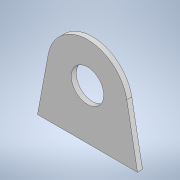
# Autodesk Inventor part: 76. Стопор штуцера
Saved by Autodesk Inventor 2021 (Build 250183000, 183)
## iProperties
Created: 2021-03-15
Part Number: 76. Стопор штуцера
Material: Типовые
Document SubType Name: Modeling
Designer: Данил
Density: 1 g/cm^3
Appearance: По умолчанию
Author: Данил
Autodesk Inventor part; units mm, degrees
ref_plane "YZ Plane" through (0, 0, 0) normal (1, 0, 0) x (0, 1, 0)
ref_plane "XZ Plane" through (0, 0, 0) normal (0, 1, 0) x (-1, 0, 0)
ref_plane "XY Plane" through (0, 0, 0) normal (0, 0, 1) x (1, 0, 0)
sketch "Эскиз1" plane through (0, 0, 0) normal (0, 0, 1) x (1, 0, 0)
  line L0 (0, 9) -> (0, -9) construction
  line L1 (0, -9) -> (10, -9)
  arc A0 (0, -2.25) -> (0, 4.25) centre (0, 1) ccw
  arc A1 (7.8648, 2.4648) -> (0, 9) centre (0, 1) ccw
  line L2 (7.8648, 2.4648) -> (10, -9)
  line L3 (0, 9) -> (0, 4.25)
  line L4 (0, -2.25) -> (0, -9)
  point P0 (0, 0)
  point P1 (0, 0)
  dimension "d0" = 18
  dimension "d1" = 10
  dimension "d2" = 3.25
  dimension "d3" = 10
  constraints: 10 end point, 4 point on circle, 3 point on line, 2 centre point, 2 coincident, 2 collinear, 1 horizontal, 1 midpoint, 1 tangent, 1 vertical
  measures "d0" distance of L0.start L0.end
  measures "d1" distance of L0.end L1.end
  measures "d2" radius of A0
  measures "d3" distance of L0.end A0.centre
extrude "Выдавливание1" add sketch "Эскиз1" along normal blind 1
mirror "Зеркальное отражение1" about plane through (0, 0, 0) normal (1, 0, 0) of "Выдавливание1"
